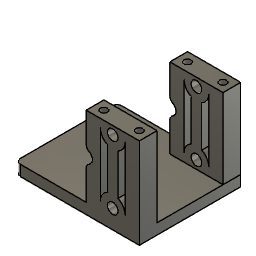
2026_05_012_archivo_fusion_360_chasis_robot_sumo_v2 (Autodesk Fusion 360 archive; units mm, degrees)
design "soporte para el motor v2"
Autodesk Fusion 360 part; units mm, degrees
sketch "Boceto1" plane through (0, 0, 0) normal (0, 0, 1) x (1, 0, 0)
  line L0 (0, 0) -> (15, 0)
  line L1 (15, 0) -> (15, 22.5)
  line L2 (15, 22.5) -> (0, 22.5)
  line L3 (0, 22.5) -> (0, 0)
  line L4 (0, 22.5) -> (7.5, 22.5)
  line L5 (7.5, 22.5) -> (7.5, 17.9)
  line L6 (7.5, 17.9) -> (7.5, 20.2)
  circle A0 centre (7.5, 20.2) radius 1.5
  line L7 (7.5, 0) -> (7.5, 4.6)
  line L8 (7.5, 0) -> (7.5, 2.3)
  circle A1 centre (7.5, 2.3) radius 1.5
  line L9 (12.6715, 2.3285) -> (12.6715, 20.1715)
  line L10 (2.3285, 20.1715) -> (2.3285, 2.3285)
  arc A2 (4.0001, 20.1715) -> (10.9999, 20.1715) centre (7.5, 20.2) ccw
  arc A3 (10.9999, 2.3285) -> (4.0001, 2.3285) centre (7.5, 2.3) ccw
  line L11 (8.9997, 20.1715) -> (8.9997, 2.3285)
  line L12 (6.0003, 2.3285) -> (6.0003, 20.1715)
  line L13 (4.0001, 20.1715) -> (2.3285, 20.1715)
  line L14 (12.6715, 20.1715) -> (10.9999, 20.1715)
  line L15 (2.3285, 2.3285) -> (6.0003, 2.3285)
  line L16 (8.9997, 2.3285) -> (12.6715, 2.3285)
  line L17 (10.9999, 20.1715) -> (10.9999, 2.3285)
  line L18 (4.0001, 20.1715) -> (4.0001, 2.3285)
  dimension "d1" = 15
  dimension "d2" = 22.5
  dimension "d3" = 7.5
  dimension "d4" = 4.6
  dimension "d5" = 2.3
  dimension "d6" = 3
  dimension "d7" = 4.6
  dimension "d8" = 2.3
  dimension "d9" = 3
  constraint horizontal L0
  constraint vertical L1
  constraint horizontal L2
  constraint vertical L3
  constraint coincident L0.start L3.end
  constraint perpendicular L3 L4
  constraint perpendicular L2 L5
  constraint parallel L5 L6
  constraint coincident L6.end A0.centre
  constraint midpoint L0 L7.start
  constraint perpendicular L0 L7
  constraint perpendicular L0 L8
  constraint coincident L8.end A1.centre
  constraint concentric A0 A2
  constraint coincident A2.start L14
  constraint concentric A1 A3
  constraint coincident A3.start L15
  constraint coincident A3.end L15
  constraint coincident A0 L11.start
  constraint coincident L11.start L14
  constraint coincident L11.end L15
  constraint coincident A1 L11.end
  constraint coincident A1 L12.start
  constraint coincident A0 L12.end
  constraint collinear L13 L14
  constraint collinear L15 L16
  constraint perpendicular L16 L17
  measures "d1" distance of L0.start L0.end
  measures "d2" distance of L0.start L2.end
  measures "d3" distance of L2.end L4.end
  measures "d4" distance of L4.end L5.end
  measures "d5" distance of L5.end L6.end
  measures "d6" diameter of A0
  measures "d7" distance of L7.start L7.end
  measures "d8" distance of L7.start L8.end
  measures "d9" diameter of A1
extrude "Extruir1" add sketch "Boceto1" along normal blind 5 contours L0 L2 L3 L4 L5 A0 L7 L8 A1 L10 A2 L12 L13 L15 | L0 L1 L2 L5 A0 L7 L8 A1 L9 A2 L11 L14 L16 | A1 A3 L11 L12 | A3 L12 L15 | A2 A3 L11 L12 | L10 L13 L15 L18 | A3 L11 L16 | A0 A2 L11 L12 | L9 L14 L16 L17
sketch "Boceto2" plane through (0, 22.5, 0) normal (0, 1, 0) x (-1, 0, 0)
  line L0 (-15, 0) -> (0, 0)
  line L1 (0, 0) -> (0, 5)
  line L2 (0, 5) -> (-15, 5)
  line L3 (-15, 5) -> (-15, 0)
  line L4 (0, 5) -> (0, 2.5)
  line L5 (0, 2.5) -> (-2.5, 2.5)
  line L6 (-2.5, 2.5) -> (-12.5, 2.5)
  line L7 (-12.5, 2.5) -> (-15, 2.5)
  circle A0 centre (-2.5, 2.5) radius 1
  circle A1 centre (-12.5, 2.5) radius 1
  dimension "d15" = 2.5
  dimension "d16" = 2.5
  dimension "d17" = 10
  dimension "d18" = 2.5
  dimension "d19" = 2
  dimension "d20" = 2
  constraint coincident L1.end L2.start
  constraint perpendicular L0 L4
  constraint perpendicular L1 L5
  constraint parallel L5 L6
  constraint parallel L6 L7
  constraint coincident L5.end L6.start
  constraint coincident L6.end L7.start
  measures "d15" distance of L1.end L4.end
  measures "d16" distance of L4.end L5.end
  measures "d17" distance of L5.end L6.end
  measures "d18" distance of L6.end L7.end
  measures "d19" diameter of A0
  measures "d20" diameter of A1
extrude "Extruir2" cut sketch "Boceto2" against normal blind 6 contours L6 L7 A1 | L6 L7 A1 | L5 L6 A0 | L5 L6 A0
extrude "Extruir3" add 1 faces at (5, 0, 1.6667) along direction (0, -1, 0) blind 3
sketch "Boceto3" plane through (0, 0, 0) normal (0, 0, -1) x (-1, 0, 0)
  circle A0 centre (-7.5, 2.3) radius 1.5
  circle A1 centre (-7.5, 20.2) radius 1.5
  line L0 (-8.9997, 17.0376) -> (-8.9997, 5.4624)
  arc A2 (-8.9997, 5.4624) -> (-10.9999, 2.3285) centre (-7.5, 2.3) ccw
  line L1 (-10.9999, 2.3285) -> (-10.9999, 20.1715)
  arc A3 (-10.9999, 20.1715) -> (-8.9997, 17.0376) centre (-7.5, 20.2) ccw
  line L2 (-6.0003, 5.4624) -> (-6.0003, 17.0376)
  arc A4 (-6.0003, 17.0376) -> (-4.0001, 20.1715) centre (-7.5, 20.2) ccw
  line L3 (-4.0001, 20.1715) -> (-4.0001, 2.3285)
  arc A5 (-4.0001, 2.3285) -> (-6.0003, 5.4624) centre (-7.5, 2.3) ccw
  line L4 (0, -3) -> (0, 22.5)
  line L5 (0, 22.5) -> (-15, 22.5)
  line L6 (-15, 22.5) -> (-15, -3)
  line L7 (-15, -3) -> (0, -3)
  line L8 (0, -3) -> (-15, -3)
  line L9 (-15, -3) -> (-15, 0)
  line L10 (-15, 0) -> (0, 0)
  line L11 (0, -3) -> (20, -3)
  line L12 (20, -3) -> (20, 0)
  line L13 (20, 0) -> (0, 0)
  dimension "d25" = 20
  constraint horizontal L8
  constraint vertical L9
  constraint horizontal L10
  constraint coincident L6 L9.end
  constraint coincident L4.start L7.end
  constraint perpendicular L4 L11
  constraint perpendicular L11 L12
  constraint perpendicular L4 L13
  measures "d25" distance of L4.start L11.end
extrude "Extruir4" add sketch "Boceto3" along normal blind 23.6 contours L4 L6 L7 L8 L9 L10 | L4 L11 L12 L13
ref_plane "PlanoDeObra1" through (-2.5, -1.5, -23.6) normal (0, 0, -1) x (-1, 0, 0)
sketch "Boceto4" plane through (0, 0, -23.6) normal (0, 0, -1) x (-1, 0, 0)
  line L0 (-10.9999, 20.1715) -> (-10.9999, 2.3285)
  line L1 (-15, 22.5) -> (-7.5, 22.5)
  line L2 (0, 22.5) -> (-15, 22.5)
  line L3 (0, 0) -> (0, 22.5)
  line L4 (-2.3285, 0) -> (0, 0)
  line L5 (-2.3285, 0) -> (-15, 0)
  line L6 (-15, 0) -> (-15, 22.5)
  circle A0 centre (-7.5, 2.3) radius 1.5
  circle A1 centre (-7.5, 20.2) radius 1.5
  line L7 (-4.0001, 2.3285) -> (-4.0001, 20.1715)
  line L8 (-10.9999, 20.1715) -> (-10.9999, 2.3285)
  line L9 (-9.0139, 17.0443) -> (-9.0139, 5.4557)
  line L10 (-5.9861, 5.4557) -> (-5.9861, 17.0443)
  arc A2 (-10.9999, 20.1715) -> (-9.0139, 17.0443) centre (-7.5, 20.2) ccw
  arc A3 (-5.9861, 17.0443) -> (-4.0001, 20.1715) centre (-7.5, 20.2) ccw
  arc A4 (-4.0001, 2.3285) -> (-5.9861, 5.4557) centre (-7.5, 2.3) ccw
  arc A5 (-9.0139, 5.4557) -> (-10.9999, 2.3285) centre (-7.5, 2.3) ccw
  point P0 (-8.9997, 20.1715)
  dimension "d29" = 7.5
  dimension "d31" = 3
  dimension "d32" = 3
  constraint vertical L3
  constraint horizontal L2
  constraint perpendicular L3 L4
  constraint concentric A1 A2
  constraint concentric A0 A4
  constraint coincident L9.end A4
  constraint vertical L9
  constraint coincident L10.end A2
  constraint parallel L9 L10
  constraint concentric A2 A3
  constraint concentric A4 A5
  measures "d29" distance of L1.start L1.end
  measures "d31" diameter of A0
  measures "d32" diameter of A1
extrude "Extruir5" add sketch "Boceto4" against normal blind 5
sketch "Boceto6" plane through (0, 22.5, 0) normal (0, 1, 0) x (-1, 0, 0)
  line L0 (-15, -23.6) -> (0, -23.6)
  line L1 (0, -23.6) -> (0, -18.6)
  line L2 (0, -18.6) -> (-15, -18.6)
  line L3 (-15, -18.6) -> (-15, -23.6)
  line L4 (0, -23.6) -> (0, -21.1)
  line L5 (0, -21.1) -> (-15, -21.1)
  line L6 (0, -23.6) -> (-2.5, -23.6)
  circle A0 centre (-2.5, -21.1) radius 1
  line L7 (-15, -23.6) -> (-12.5, -23.6)
  circle A1 centre (-12.4985, -21.1) radius 1
  dimension "d35" = 15
  dimension "d36" = 2.5
  dimension "d37" = 2.5
  dimension "d38" = 2
  dimension "d39" = 2.5
  dimension "d40" = 2
  constraint coincident L0.end L1.start
  constraint midpoint L1 L4.end
  constraint midpoint L3 L5.end
  constraint perpendicular L4 L6
  constraint coincident L5 A0.centre
  constraint coincident L0.start L3.end
  constraint perpendicular L3 L7
  constraint coincident L5 A1.centre
  measures "d35" distance of L4.end L5.end
  measures "d36" distance of L0.end L4.end
  measures "d37" distance of L0.end L6.end
  measures "d38" diameter of A0
  measures "d39" distance of L0.start L7.end
  measures "d40" diameter of A1
extrude "Extruir6" cut sketch "Boceto6" against normal blind 6 contours L5 A1 | L5 A1 | L5 A0 | L5 A0
extrude "Extruir7" add 1 faces at (-6.6667, -1, 0) along direction (0, 0, 1) blind 5
sketch "Boceto7" plane through (0, 0, 0) normal (0, 0, 1) x (1, 0, 0)
  line L0 (0, 0) -> (0, 22.5)
  line L1 (0, 11.25) -> (-2, 11.25)
  circle A0 centre (0, 11.25) radius 1.75
  dimension "d45" = 22.5
  dimension "d46" = 3.5
  constraint coincident L0.start origin
  constraint vertical L0
  constraint midpoint L0 L1.start
  constraint perpendicular L0 L1
  constraint coincident L1.start A0.centre
  measures "d45" distance of L0.start L0.end
  measures "d46" diameter of A0
extrude "Extruir8" cut sketch "Boceto7" along normal mid plane 68
fillet "Empalme1" radius 1.5 4 edges at (0, 9.5, -21.1) (0, 13, -21.1) (0, 9.5, 2.5) (0, 13, 2.5)
fillet "Empalme2" radius 1.5 2 edges at (-20, -1.5, 5) (-20, -1.5, -23.6)

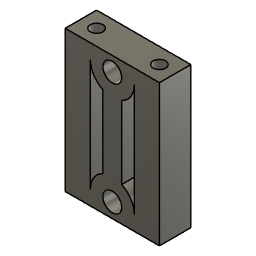
design "soporte para el motor"
Autodesk Fusion 360 part; units mm, degrees
sketch "Boceto1" plane through (0, 0, 0) normal (0, 0, 1) x (1, 0, 0)
  line L0 (0, 0) -> (15, 0)
  line L1 (15, 0) -> (15, 22.5)
  line L2 (15, 22.5) -> (0, 22.5)
  line L3 (0, 22.5) -> (0, 0)
  line L4 (0, 22.5) -> (7.5, 22.5)
  line L5 (7.5, 22.5) -> (7.5, 17.9)
  line L6 (7.5, 17.9) -> (7.5, 20.2)
  circle A0 centre (7.5, 20.2) radius 1.5
  line L7 (7.5, 0) -> (7.5, 4.6)
  line L8 (7.5, 0) -> (7.5, 2.3)
  circle A1 centre (7.5, 2.3) radius 1.5
  line L9 (12.6715, 2.3285) -> (12.6715, 20.1715)
  line L10 (2.3285, 20.1715) -> (2.3285, 2.3285)
  arc A2 (4.0001, 20.1715) -> (10.9999, 20.1715) centre (7.5, 20.2) ccw
  arc A3 (10.9999, 2.3285) -> (4.0001, 2.3285) centre (7.5, 2.3) ccw
  line L11 (8.9997, 20.1715) -> (8.9997, 2.3285)
  line L12 (6.0003, 2.3285) -> (6.0003, 20.1715)
  line L13 (4.0001, 20.1715) -> (2.3285, 20.1715)
  line L14 (12.6715, 20.1715) -> (10.9999, 20.1715)
  line L15 (2.3285, 2.3285) -> (6.0003, 2.3285)
  line L16 (8.9997, 2.3285) -> (12.6715, 2.3285)
  line L17 (10.9999, 20.1715) -> (10.9999, 2.3285)
  line L18 (4.0001, 20.1715) -> (4.0001, 2.3285)
  dimension "d1" = 15
  dimension "d2" = 22.5
  dimension "d3" = 7.5
  dimension "d4" = 4.6
  dimension "d5" = 2.3
  dimension "d6" = 3
  dimension "d7" = 4.6
  dimension "d8" = 2.3
  dimension "d9" = 3
  constraint horizontal L0
  constraint vertical L1
  constraint horizontal L2
  constraint vertical L3
  constraint coincident L0.start L3.end
  constraint perpendicular L3 L4
  constraint perpendicular L2 L5
  constraint parallel L5 L6
  constraint coincident L6.end A0.centre
  constraint midpoint L0 L7.start
  constraint perpendicular L0 L7
  constraint perpendicular L0 L8
  constraint coincident L8.end A1.centre
  constraint concentric A0 A2
  constraint coincident A2.start L14
  constraint concentric A1 A3
  constraint coincident A3.start L15
  constraint coincident A3.end L15
  constraint coincident A0 L11.start
  constraint coincident L11.start L14
  constraint coincident L11.end L15
  constraint coincident A1 L11.end
  constraint coincident A1 L12.start
  constraint coincident A0 L12.end
  constraint collinear L13 L14
  constraint collinear L15 L16
  constraint perpendicular L16 L17
  measures "d1" distance of L0.start L0.end
  measures "d2" distance of L0.start L2.end
  measures "d3" distance of L2.end L4.end
  measures "d4" distance of L4.end L5.end
  measures "d5" distance of L5.end L6.end
  measures "d6" diameter of A0
  measures "d7" distance of L7.start L7.end
  measures "d8" distance of L7.start L8.end
  measures "d9" diameter of A1
extrude "Extruir1" add sketch "Boceto1" along normal blind 5 contours L0 L2 L3 L4 L5 A0 L7 L8 A1 L10 A2 L12 L13 L15 | L0 L1 L2 L5 A0 L7 L8 A1 L9 A2 L11 L14 L16 | A1 A3 L11 L12 | A3 L12 L15 | A2 A3 L11 L12 | L10 L13 L15 L18 | A3 L11 L16 | A0 A2 L11 L12 | L9 L14 L16 L17
sketch "Boceto2" plane through (0, 22.5, 0) normal (0, 1, 0) x (-1, 0, 0)
  line L0 (-15, 0) -> (0, 0)
  line L1 (0, 0) -> (0, 5)
  line L2 (0, 5) -> (-15, 5)
  line L3 (-15, 5) -> (-15, 0)
  line L4 (0, 5) -> (0, 2.5)
  line L5 (0, 2.5) -> (-2.5, 2.5)
  line L6 (-2.5, 2.5) -> (-12.5, 2.5)
  line L7 (-12.5, 2.5) -> (-15, 2.5)
  circle A0 centre (-2.5, 2.5) radius 1
  circle A1 centre (-12.5, 2.5) radius 1
  dimension "d15" = 2.5
  dimension "d16" = 2.5
  dimension "d17" = 10
  dimension "d18" = 2.5
  dimension "d19" = 2
  dimension "d20" = 2
  constraint coincident L1.end L2.start
  constraint perpendicular L0 L4
  constraint perpendicular L1 L5
  constraint parallel L5 L6
  constraint parallel L6 L7
  constraint coincident L5.end L6.start
  constraint coincident L6.end L7.start
  measures "d15" distance of L1.end L4.end
  measures "d16" distance of L4.end L5.end
  measures "d17" distance of L5.end L6.end
  measures "d18" distance of L6.end L7.end
  measures "d19" diameter of A0
  measures "d20" diameter of A1
extrude "Extruir2" cut sketch "Boceto2" against normal blind 6 contours L6 L7 A1 | L6 L7 A1 | L5 L6 A0 | L5 L6 A0
